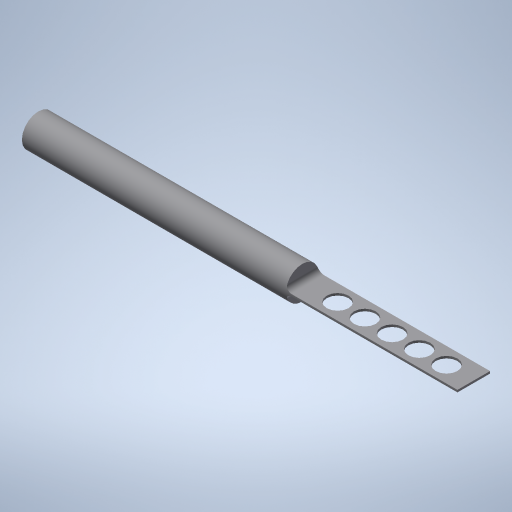
# Autodesk Inventor part: 5_multi_beetle_holder
Saved by Autodesk Inventor 2023.2 (Build 272271000, 271)
## iProperties
Created: 2022-10-21
Part Number: 5_multi_beetle_holder
Material: Generisch
Document SubType Name: Modeling
Designer: splath
Density: 1 g/cm^3
Appearance: Vorgabe
Author: splath
Autodesk Inventor part; units mm, degrees
ref_plane "YZ Plane" through (0, 0, 0) normal (1, 0, 0) x (0, 1, 0)
sketch "Sketch1" plane through (0, 0, 0) normal (1, 0, 0) x (0, 1, 0)
  circle A0 centre (0, 0) radius 1.5
  dimension "d0" = 3
  constraints: 1 centre point, 1 coincident
  measures "d0" diameter of A0
extrude "Extrusion1" add sketch "Sketch1" along normal blind 71
ref_plane "Work Plane1" through (0, 0, -1.5) normal (0, 0, 1) x (1, 0, 0)
sketch "Sketch3" plane through (0, 0, -1.5) normal (0, 0, 1) x (1, 0, 0)
  line L0 (-14.2, 0) -> (85.2, 0) construction
  line L1 (0, -1.5) -> (0, 1.5) construction
  point P0 (0, 0)
  point P1 (27.5, 0)
  dimension "d16" = 27.5
  constraints: 1 point on line
  measures "d16" distance from line of L1 point (27.5, 0)
hole "Hole1" at (27.5, 0, -1.5) direction (0, 0, 1) diameter 2 end through all
pattern_linear "Rectangular Pattern1" count 5 spacing 2.5 along (1, 0, 0) of "Hole1"
sketch "Sketch2" plane through (0, 0, 0) normal (0, 1, 0) x (-1, 0, 0)
  line L0 (-71, 1.5) -> (-71, -1.5) construction
  line L1 (0, 1.5) -> (0, -1.5) construction
  line L2 (-24.25, 1.5) -> (-40.75, 1.5)
  line L3 (-40.75, 1.5) -> (-40.75, 0.6)
  line L4 (-40.25, 0.1) -> (-24.75, 0.1)
  line L5 (-24.25, 0.6) -> (-24.25, 1.5)
  line L6 (-24.25, -1.5) -> (-40.75, -1.5)
  line L7 (-40.75, -1.5) -> (-40.75, -0.6)
  line L8 (-40.25, -0.1) -> (-24.75, -0.1)
  line L9 (-24.25, -0.6) -> (-24.25, -1.5)
  line L10 (0, 1.5) -> (-71, 1.5) construction
  line L11 (0, -1.5) -> (-71, -1.5) construction
  line L12 (13.2, 0) -> (-79.2, 0) construction
  arc A0 (-24.75, 0.1) -> (-24.25, 0.6) centre (-24.75, 0.6) ccw
  arc A1 (-40.75, 0.6) -> (-40.25, 0.1) centre (-40.25, 0.6) ccw
  arc A2 (-24.25, -0.6) -> (-24.75, -0.1) centre (-24.75, -0.6) ccw
  arc A3 (-40.25, -0.1) -> (-40.75, -0.6) centre (-40.25, -0.6) ccw
  point P0 (0, 0)
  dimension "d3" = 0.5
  dimension "d4" = 0.2
  dimension "d20" = 16.5
  dimension "d21" = 24.25
  constraints: 16 end point, 8 point on circle, 8 tangent, 4 centre point, 4 collinear, 4 parallel, 3 equal radius, 2 horizontal, 2 perpendicular, 1 other
  measures "d3" radius of A0
  measures "d4" distance between parallel lines of L8 L4
  measures "d20" distance of L2.start L2.end
  measures "d21" distance between parallel lines of L1 L5
extrude "Extrusion2" cut sketch "Sketch2" along normal through all both and the other way through all
ref_plane "Work Plane2" through (0, 0, 0) normal (0, 0.7071, 0.7071) x (1, 0, 0)
sketch "Sketch4" plane through (0, 0, 0) normal (0, 0.7071, 0.7071) x (1, 0, 0)
  line L0 (26.9374, -0.3516) -> (28.0626, -0.3516)
  line L1 (28.0626, -0.3516) -> (28.0626, 0.3516)
  line L2 (28.0626, 0.3516) -> (26.9374, 0.3516)
  line L3 (26.9374, 0.3516) -> (26.9374, -0.3516)
  line L4 (26.9374, -0.3516) -> (28.0626, 0.3516) construction
  line L5 (28.0626, -0.3516) -> (26.9374, 0.3516) construction
  line L6 (26.7934, -0.5175) -> (28.2066, -0.5175)
  line L7 (28.2066, -0.5175) -> (28.2066, 0.5175)
  line L8 (28.2066, 0.5175) -> (26.7934, 0.5175)
  line L9 (26.7934, 0.5175) -> (26.7934, -0.5175)
  line L10 (26.7934, -0.5175) -> (28.2066, 0.5175) construction
  line L11 (28.2066, -0.5175) -> (26.7934, 0.5175) construction
  line L12 (27.1467, -0.2588) -> (27.8533, -0.2588)
  line L13 (27.8533, -0.2588) -> (27.8533, 0.2587)
  line L14 (27.8533, 0.2587) -> (27.1467, 0.2587)
  line L15 (27.1467, 0.2587) -> (27.1467, -0.2588)
  line L16 (27.1467, -0.2588) -> (27.8533, 0.2587) construction
  line L17 (27.8533, -0.2588) -> (27.1467, 0.2587) construction
  line L18 (-5.7, 0) -> (34.2, 0) construction
  ellipse E0 centre (27.5, -0.0707) end of major axis (28.5, -0.0707) minor radius 0.7071 construction
  ellipse E1 centre (27.5, 0.0707) end of major axis (28.5, 0.0707) minor radius 0.7071 construction
  line L19 (27.5, -0.0707) -> (27.5, 0.0707) construction
  point P0 (0, 0)
  point P1 (27.5, 0)
  dimension "d23" = 0.7032
  dimension "d24" = 1.1251
  dimension "d25" = 1.4131
  dimension "d26" = 1.035
  dimension "d27" = 0.5175
  dimension "d28" = 0.7066
  constraints: 38 end point, 7 midpoint, 6 parallel, 3 horizontal, 3 perpendicular, 1 vertical
  measures "d23" distance of L1.start L1.end
  measures "d24" distance of L1.end L2.end
  measures "d25" distance of L11.end L8.start
  measures "d26" distance of L6.end L8.start
  measures "d27" distance of L12.end L13.end
  measures "d28" distance of L15.end L12.end
sketch "Sketch5" plane through (71, 0, 0) normal (1, 0, 0) x (0, 0, -1)
  circle A0 centre (0, 0) radius 1.5 projected
extrude "Extrusion3" cut sketch "Sketch5" against normal blind 31
equation "\"d16\" = DistanceHoleEnd"
equation "\"d9\" = DiameterHole"
equation "\"d19\" = DistanceHoleHole"
equation "\"d4\" = Thickness"
equation "\"DistanceHoleHole\" = 2.5"
equation "\"DiameterHole\" = 2"
equation "\"DistanceHoleEnd\" = 27.5"
equation "\"Thickness\" = 0.2"
body "Solid1"
